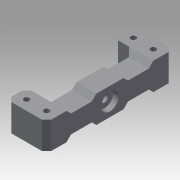
# Autodesk Inventor part: Wheel_Block
Saved by Autodesk Inventor 2016 (Build 200138000, 138)
## iProperties
Created: 2015-06-05
Part Number: Wheel_Block
Material: Générique
Document SubType Name: Modeling
Designer: Logan
Density: 1 g/cm^3
Appearance: Par défaut
Author: Logan
Autodesk Inventor part; units mm, degrees
note: some values were not read from the file. Chosen so that the rebuilt part matches the saved one: sketch regions of "Extrusion19".
ref_plane "YZ Plane" through (0, 0, 0) normal (1, 0, 0) x (0, 1, 0)
ref_plane "XZ Plane" through (0, 0, 0) normal (0, 1, 0) x (-1, 0, 0)
ref_plane "XY Plane" through (0, 0, 0) normal (0, 0, 1) x (1, 0, 0)
sketch "Esquisse17" plane through (0, 0, 0) normal (0, 0, 1) x (1, 0, 0)
  line L0 (-22, 70) -> (22, 70)
  line L1 (22, 70) -> (22, -70)
  line L2 (22, -70) -> (-22, -70)
  line L3 (-22, -70) -> (-22, 70)
  point P0 (0, 0)
  dimension "d107" = 70
  dimension "d108" = 140
  dimension "d109" = 44
  dimension "d110" = 22
  constraints: 8 end point, 2 parallel, 1 horizontal, 1 perpendicular
  measures "d107" distance from line of L2 point (0, 0)
  measures "d108" distance of L0.end L1.end
  measures "d109" distance between parallel lines of L1 L3
  measures "d110" distance from line of point (0, 0) L3
extrude "Extrusion13" add sketch "Esquisse17" along normal mid plane 30
sketch "Esquisse18" plane through (22, -70, 15) normal (1, 0, 0) x (0, 0, -1)
  circle A0 centre (15, 70) radius 4
  dimension "d113" = 8
  constraints: 1 centre point, 1 coincident
  measures "d113" diameter of A0
extrude "Extrusion14" cut sketch "Esquisse18" against normal up to next
sketch "Esquisse19" plane through (22, -70, 15) normal (1, 0, 0) x (0, 0, -1)
  circle A0 centre (15, 70) radius 9.5
  dimension "d116" = 19
  constraints: 1 centre point, 1 coincident
  measures "d116" diameter of A0
extrude "Extrusion15" cut sketch "Esquisse19" against normal blind 6
sketch "Esquisse20" plane through (0, 0, 15) normal (0, 0, 1) x (1, 0, 0)
  line L0 (-22, 48) -> (0, 48)
  line L1 (0, 48) -> (0, -48)
  line L2 (0, -48) -> (-22, -48)
  line L3 (-22, -48) -> (-22, 48)
  line L4 (22, -70) -> (22, 70) projected
  line L5 (-22, 70) -> (-22, -70) projected
  point P0 (0, 0)
  dimension "d119" = 96
  dimension "d120" = 48
  dimension "d121" = 22
  constraints: 8 end point, 2 parallel, 1 collinear, 1 horizontal, 1 perpendicular
  measures "d119" distance between parallel lines of L2 L0
  measures "d120" distance from line of point (0, 0) L0
  measures "d121" distance between parallel lines of L4 L1
extrude "Extrusion16" cut sketch "Esquisse20" against normal up to next
sketch "Esquisse21" plane through (0, -48, 15) normal (-1, 0, 0) x (0, 0, 1)
  circle A0 centre (-15, 48) radius 9.5
  dimension "d125" = 19
  constraints: 1 centre point, 1 coincident
  measures "d125" diameter of A0
extrude "Extrusion17" cut sketch "Esquisse21" against normal blind 6
sketch "Esquisse22" plane through (22, -70, 15) normal (1, 0, 0) x (0, 0, -1)
  line L0 (5, 0) -> (25, 0)
  line L1 (25, 140) -> (5, 140)
  line L2 (0, 0) -> (30, 0) projected
  line L3 (0, 140) -> (30, 140) projected
  line L4 (0, 0) -> (0, 140) projected
  line L5 (30, 140) -> (30, 0) projected
  line L6 (30, 55) -> (30, 85)
  line L7 (0, 85) -> (0, 55)
  line L8 (0, 55) -> (0, 55)
  line L9 (30, 55) -> (30, 55)
  line L10 (5, 140) -> (5, 90)
  line L11 (5, 50) -> (5, 0)
  line L12 (25, 0) -> (25, 50)
  line L13 (25, 90) -> (25, 140)
  line L14 (30, 85) -> (30, 85)
  line L15 (0, 85) -> (0, 85)
  line L16 (0, 55) -> (5, 50)
  line L17 (5, 90) -> (0, 85)
  line L18 (25, 90) -> (30, 85)
  line L19 (30, 55) -> (25, 50)
  line L20 (0, 118) -> (5, 118)
  line L21 (25, 118) -> (30, 118)
  line L22 (0, 22) -> (5, 22)
  line L23 (25, 22) -> (30, 22)
  point P0 (15, 70)
  point P1 (5, 55)
  point P2 (25, 55)
  point P3 (5, 85)
  point P4 (25, 85)
  dimension "d131" = 30
  dimension "d133" = 20
  dimension "d134" = 10
  dimension "d135" = 30
  dimension "d136" = 15
  dimension "d137" = 5
  dimension "d138" = 5
  dimension "d139" = 5
  dimension "d140" = 5
  dimension "d141" = 5
  dimension "d142" = 5
  dimension "d143" = 5
  dimension "d144" = 5
  constraints: 40 end point, 12 point on line, 10 parallel, 8 collinear, 4 perpendicular, 3 horizontal
  measures "d131" distance of L2.start L2.end
  measures "d133" distance between parallel lines of L12 L11
  measures "d134" distance from line of point (15, 70) L11
  measures "d135" distance between parallel lines of L15 L8
  measures "d136" distance from line of point (15, 70) L15
  measures "d137" distance of L8.end point (5, 55)
  measures "d138" distance of L11.start point (5, 55)
  measures "d139" distance of L10.end point (5, 85)
  measures "d140" distance of L15.start point (5, 85)
  measures "d141" distance of L13.start point (25, 85)
  measures "d142" distance of L14.end point (25, 85)
  measures "d143" distance of L9.start point (25, 55)
  measures "d144" distance of L12.end point (25, 55)
extrude "Extrusion19" cut sketch "Esquisse22" against normal up to next contours L22 L4 L16 L11 | L12 L19 L5 L23 | L4 L20 L10 L17 | L18 L13 L21 L5
chamfer "Chanfrein3" distance 5 angle 45 10 edges at (11, -48, -10) (11, -48, 10) (11, 48, 10) (11, 48, -10) (-22, -48, 0) (-22, -70, 0) (-22, 48, 0) (-22, 70, 0) (22, -70, 0) (22, 70, 0)
sketch "Esquisse23" plane through (0, 0, -15) normal (0, 0, -1) x (-1, 0, 0)
  line L0 (-11, -59) -> (11, -59)
  line L1 (17, -48) -> (0, -48) projected
  line L2 (0, -48) -> (-22, -48) projected
  line L3 (-22, -48) -> (-22, -65) projected
  line L4 (-17, -70) -> (17, -70) projected
  line L5 (22, -65) -> (22, -53) projected
  line L6 (-46.7579, 0) -> (65.4048, 0)
  line L7 (-11, 59) -> (11, 59)
  line L8 (20, 48) -> (0, 48)
  line L9 (0, 48) -> (-22, 48)
  line L10 (-22, 48) -> (-22, 70)
  line L11 (-22, 70) -> (20, 70)
  line L12 (20, 70) -> (20, 48)
  line L13 (0, 15) -> (-22, 15) projected
  line L14 (-22, 15) -> (-22, -15) projected
  line L15 (-22, -15) -> (0, -15) projected
  line L16 (0, -15) -> (0, 15) projected
  line L17 (-17, -70) -> (-22, -65) projected
  line L18 (22, -65) -> (17, -70) projected
  line L19 (17, -48) -> (22, -53) projected
  line L20 (-22, 65) -> (-17, 70) projected
  line L21 (-22, 48) -> (0, 48) projected
  line L22 (0, 48) -> (17, 48) projected
  line L23 (22, 53) -> (17, 48) projected
  line L24 (22, 53) -> (22, 65) projected
  line L25 (17, 70) -> (22, 65) projected
  line L26 (17, 70) -> (-17, 70) projected
  line L27 (-22, 65) -> (-22, 48) projected
  point P0 (0, 0)
  dimension "d153" = 11
  dimension "d154" = 11
  dimension "d155" = 11
  constraints: 16 end point, 4 symmetric about line, 2 horizontal
  measures "d153" distance between parallel lines of L4 L0
  measures "d154" distance from line of L5 L0.end
  measures "d155" distance from line of L3 L0.start
hole "Perçage4" at (11, -59, -15) at (-11, -59, -15) at (11, 59, -15) at (-11, 59, -15) direction (0, 0, 1) diameter 6 end through all counterbore diameter 10 counterbore depth 4
chamfer "Chanfrein4" distance 5 angle 45 2 edges at (0, 48, 0) (0, -48, 0)
equation "\"d107\" = 0.5 * d108"
equation "\"d110\" = 0.5 * d109"
equation "\"d120\" = 0.5 * d119"
equation "\"d134\" = 0.5 * d133"
equation "\"d135\" = d131"
equation "\"d136\" = 0.5 * d135"
equation "\"d138\" = d137"
equation "\"d139\" = d137"
equation "\"d140\" = d139"
equation "\"d141\" = d137"
equation "\"d142\" = d141"
equation "\"d143\" = d137"
equation "\"d144\" = d143"
equation "\"d153\" = 0.5 * d152"
equation "\"d154\" = d153"
equation "\"d155\" = d153"
equation "\"d132\" = 0.5 * d130"
equation "\"d152\" = 22"
equation "\"d130\" = 30"
